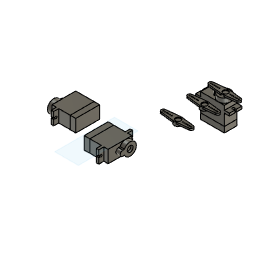
Chassis v8 (Autodesk Fusion 360 archive; units mm, degrees)
design "servo"
Autodesk Fusion 360 part; units mm, degrees
sketch "Sketch1" plane through (0, 0, 0) normal (0, 0, 1) x (1, 0, 0)
  line L0 (16, -5.9) -> (-16, -5.9)
  line L1 (-16, -5.9) -> (-16, 5.9)
  line L2 (-16, 5.9) -> (16, 5.9)
  line L3 (16, 5.9) -> (16, -5.9)
  line L4 (16, -5.9) -> (-16, 5.9) construction
  line L5 (-16, -5.9) -> (16, 5.9) construction
  line L6 (0, 0) -> (0, -5.9)
  circle A0 centre (-13.9, 0) radius 1.05
  line L7 (0, 0) -> (-16, 0)
  line L8 (-16, -0.575) -> (-14.7786, -0.575)
  line L9 (-16, 0.575) -> (-14.7786, 0.575)
  line L10 (16, -0.575) -> (14.7786, -0.575)
  circle A1 centre (13.9, 0) radius 1.05
  line L11 (16, 0.575) -> (14.7786, 0.575)
  dimension "d1" = 32
  dimension "d2" = 11.8
  dimension "d3" = 2.1
  dimension "d4" = 2.1
  dimension "d5" = 0.575
  constraint horizontal L0
  constraint perpendicular L0 L1
  constraint parallel L0 L2
  constraint parallel L1 L3
  constraint coincident L4 L6.start
  constraint coincident L5 L6.start
  constraint coincident L6.start L7.start
  constraint midpoint L0 L6.end
  constraint midpoint L1 L7.end
  constraint coincident L1 L8.start
  constraint coincident A0 L8.end
  constraint perpendicular L1 L8
  constraint coincident A0.centre L7
  constraint symmetric L7 L8.start L9.start
  constraint symmetric L7 L8.end L9.end
  constraint symmetric L6 A0 A1
  constraint symmetric L6 L8.start L10.start
  constraint symmetric L6 L8.end L10.end
  constraint symmetric L6 L9.start L11.start
  constraint symmetric L6 L9.end L11.end
  measures "d1" distance of L1.end L2.end
  measures "d2" distance of L0.end L1.end
  measures "d3" diameter of A0
  measures "d4" distance of L1 A0.centre
  measures "d5" distance of L7 L8
extrude "Extrude1" add sketch "Sketch1" along normal blind 2.3 contours L0 L1 L2 L3 L6 A0 L7 L9 L10 A1 L11 | L0 L1 L6 A0 L7 L8 makes body 1
sketch "Sketch2" plane through (0, 0, 2.3) normal (0, 0, 1) x (-1, 0, 0)
  line L0 (16, -0.575) -> (14.7786, -0.575)
  arc A0 (14.7786, 0.575) -> (14.7786, -0.575) centre (13.9, 0) ccw
  line L1 (14.7786, 0.575) -> (16, 0.575)
  line L2 (16, 0.575) -> (16, 5.9)
  line L3 (16, 5.9) -> (-16, 5.9)
  line L4 (-16, 5.9) -> (-16, 0.575)
  line L5 (-16, 0.575) -> (-14.7786, 0.575)
  arc A1 (-14.7786, -0.575) -> (-14.7786, 0.575) centre (-13.9, 0) ccw
  line L6 (-14.7786, -0.575) -> (-16, -0.575)
  line L7 (-16, -0.575) -> (-16, -5.9)
  line L8 (-16, -5.9) -> (16, -5.9)
  line L9 (16, -5.9) -> (16, -0.575)
  line L10 (11.25, -5.9) -> (-11.25, -5.9)
  line L11 (-11.25, -5.9) -> (-11.25, 5.9)
  line L12 (-11.25, 5.9) -> (11.25, 5.9)
  line L13 (11.25, 5.9) -> (11.25, -5.9)
  line L14 (11.25, -5.9) -> (-11.25, 5.9) construction
  line L15 (-11.25, -5.9) -> (11.25, 5.9) construction
  dimension "d8" = 22.5
  constraint horizontal L10
  constraint perpendicular L10 L11
  constraint parallel L10 L12
  constraint parallel L11 L13
  constraint coincident L14 origin
  constraint coincident L15 origin
  constraint coincident L3 L12.end
  measures "d8" distance of L11.end L12.end
extrude "Extrude2" add sketch "Sketch2" along normal blind 4.1 contours L3 L8 L10 L11 L12 L13 bodies 1
sketch "Sketch3" plane through (0, 0, 6.4) normal (0, 0, 1) x (-1, 0, 0)
  line L0 (11.25, 5.9) -> (-11.25, 5.9)
  line L1 (-11.25, 5.9) -> (-11.25, -5.9)
  line L2 (-11.25, -5.9) -> (11.25, -5.9)
  line L3 (11.25, -5.9) -> (11.25, 5.9)
  line L4 (0, 0) -> (-25, 0)
  line L5 (1.5394, 2.5) -> (-0.0028, 2.4935)
  line L6 (1.5394, -2.5) -> (-0.0028, -2.4935)
  arc A0 (1.5394, -2.5) -> (1.5394, 2.5) centre (1.55, 0) ccw
  arc A1 (-0.0028, 2.4935) -> (-0.0028, -2.4935) centre (-5.35, 0) ccw
  dimension "d11" = 5
  dimension "d12" = 6.9
  constraint coincident L4.start origin
  constraint parallel L0 L4
  constraint tangent L0 A1
  constraint tangent L1 A1
  constraint tangent L2 A1
  constraint tangent L5 A0
  constraint symmetric L4 L5.start L6.start
  measures "d11" diameter of A0
  measures "d12" distance of A1.centre A0.centre
extrude "Extrude3" add sketch "Sketch3" along normal blind 4.2 contours L5 L6 A0 A1 bodies 1
sketch "Sketch4" plane through (0, 0, 0) normal (0, 0, -1) x (1, 0, 0)
  line L0 (-14.7786, -0.575) -> (-16, -0.575)
  line L1 (-16, -0.575) -> (-16, -5.9)
  line L2 (-16, -5.9) -> (16, -5.9)
  line L3 (16, -5.9) -> (16, -0.575)
  line L4 (16, -0.575) -> (14.7786, -0.575)
  arc A0 (14.7786, 0.575) -> (14.7786, -0.575) centre (13.9, 0) ccw
  line L5 (14.7786, 0.575) -> (16, 0.575)
  line L6 (16, 0.575) -> (16, 5.9)
  line L7 (16, 5.9) -> (-16, 5.9)
  line L8 (-16, 5.9) -> (-16, 0.575)
  line L9 (-16, 0.575) -> (-14.7786, 0.575)
  arc A1 (-14.7786, -0.575) -> (-14.7786, 0.575) centre (-13.9, 0) ccw
  line L10 (11.25, -5.9) -> (11.25, 5.9)
  line L11 (11.25, 5.9) -> (-11.25, 5.9)
  line L12 (-11.25, 5.9) -> (-11.25, -5.9)
  line L13 (-11.25, -5.9) -> (11.25, -5.9)
extrude "Extrude4" add sketch "Sketch4" along normal blind 10.9 contours L2 L7 L10 L11 L12 L13 bodies 1
sketch "Sketch5" plane through (0, 0, -10.9) normal (0, 0, -1) x (1, 0, 0)
  line L0 (-11.25, -5.9) -> (11.25, -5.9)
  line L1 (11.25, -5.9) -> (11.25, 5.9)
  line L2 (11.25, 5.9) -> (-11.25, 5.9)
  line L3 (-11.25, 5.9) -> (-11.25, -5.9)
extrude "Extrude5" add sketch "Sketch5" along normal blind 5.3 draft 0.75 bodies 1
sketch "Sketch6" plane through (0, 0, 10.6) normal (0, 0, 1) x (-1, 0, 0)
  arc A0 (1.5394, -2.5) -> (1.5394, 2.5) centre (1.55, 0) ccw
  line L0 (1.5394, 2.5) -> (-0.0028, 2.4935)
  arc A1 (-0.0028, 2.4935) -> (-0.0028, -2.4935) centre (-5.35, 0) ccw
  line L1 (-0.0028, -2.4935) -> (1.5394, -2.5)
  circle A2 centre (-6.5803, -0.002) radius 3.58
  line L2 (-5.7591, -7.882) -> (-5.7591, 11) construction
  line L3 (-15, -0.002) -> (12, -0.002) construction
  line L4 (7.6454, 1.9853) -> (-6.1763, 3.5552)
  line L5 (7.6454, -1.9892) -> (-6.1763, -3.5591)
  circle A3 centre (7.4197, -0.002) radius 0.5
  circle A4 centre (5.8197, -0.002) radius 0.5
  circle A5 centre (4.2197, -0.002) radius 0.5
  circle A6 centre (2.6197, -0.002) radius 0.5
  circle A7 centre (1.0197, -0.002) radius 0.5
  circle A8 centre (-0.5803, -0.002) radius 0.5
  circle A9 centre (-10.9379, -0.002) radius 0.5
  circle A10 centre (-12.5379, -0.002) radius 0.5
  circle A11 centre (-14.1379, -0.002) radius 0.5
  circle A12 centre (-15.7379, -0.002) radius 0.5
  circle A13 centre (-17.3379, -0.002) radius 0.5
  circle A14 centre (-18.9379, -0.002) radius 0.5
  line L6 (-19.1636, -1.9892) -> (-5.3419, -3.5591)
  line L7 (-19.1636, 1.9853) -> (-5.3419, 3.5552)
  arc A15 (7.6454, -1.9892) -> (7.6454, 1.9853) centre (7.4197, -0.002) ccw
  arc A16 (-19.1636, 1.9853) -> (-19.1636, -1.9892) centre (-18.9379, -0.002) ccw
  dimension "d19" = 7.16
  dimension "d21" = 14
  dimension "d22" = 1
  dimension "d25" = -8
  dimension "d26" = 0
  constraint vertical L2
  constraint horizontal L3
  constraint coincident A2.centre L3
  constraint coincident A2 L4.end
  constraint tangent A2 L4
  constraint symmetric L3 L4.start L5.start
  constraint symmetric L3 L4.end L5.end
  constraint symmetric L2 L4.start L7.start
  constraint symmetric L2 L4.end L7.end
  constraint symmetric L2 L5.start L6.start
  constraint symmetric L2 L5.end L6.end
  constraint symmetric L2 A3 A14
  constraint symmetric L2 A4 A13
  constraint symmetric L2 A5 A12
  constraint symmetric L2 A6 A11
  constraint symmetric L2 A7 A10
  constraint symmetric L2 A8 A9
  measures "d19" diameter of A2
  measures "d21" distance of A2.centre A3.centre
  measures "d22" diameter of A3
extrude "Extrude6" add sketch "Sketch6" along normal blind 1.6 separate body contours A0 L0 A1 L1 A2 L4 L5 A5 L6 L7 | A0 L0 A1 L1 L4 L5 A5 A15 | A1 A9 L6 L7 A16 | A1 A2 A9 L6 L7 | A2 L6 | A2 L6 L7 | A2 L7 makes body 2
sketch "Sketch7" plane through (0, 0, 10.6) normal (0, 0, -1) x (1, 0, 0)
  circle A0 centre (18.9379, -0.002) radius 0.5
  circle A1 centre (17.3379, -0.002) radius 0.5
  circle A2 centre (-7.4197, -0.002) radius 0.5
  circle A3 centre (-5.8197, -0.002) radius 0.5
  circle A4 centre (10.9379, -0.002) radius 0.5
  circle A5 centre (15.7379, -0.002) radius 0.5
  circle A6 centre (14.1379, -0.002) radius 0.5
  circle A7 centre (-4.2197, -0.002) radius 0.5
  circle A8 centre (0.5803, -0.002) radius 0.5
  circle A9 centre (-1.0197, -0.002) radius 0.5
  circle A10 centre (-2.6197, -0.002) radius 0.5
  circle A11 centre (12.5379, -0.002) radius 0.5
  arc A12 (8.0932, 3.2427) -> (5.8336, 3.4993) centre (6.5803, -0.002) ccw
  line L0 (5.8336, 3.4993) -> (5.7591, 3.5078)
  line L1 (5.7591, 3.5078) -> (-7.6454, 1.9853)
  arc A13 (-7.6454, 1.9853) -> (-7.6454, -1.9892) centre (-7.4197, -0.002) ccw
  line L2 (-7.6454, -1.9892) -> (5.7591, -3.5117)
  line L3 (5.7591, -3.5117) -> (5.8336, -3.5032)
  arc A14 (5.8336, -3.5032) -> (8.0932, -3.2466) centre (6.5803, -0.002) ccw
  line L4 (8.0932, -3.2466) -> (19.1636, -1.9892)
  arc A15 (19.1636, -1.9892) -> (19.1636, 1.9853) centre (18.9379, -0.002) ccw
  line L5 (19.1636, 1.9853) -> (8.0932, 3.2427)
  circle A16 centre (6.5803, -0.002) radius 3.58
  constraint concentric A12 A16
  constraint tangent A12 A16
extrude "Extrude7" add sketch "Sketch7" along normal blind 1.83 contours A12 A14 A16 bodies 2
sketch "Sketch8" plane through (0, 0, 12.2) normal (0, 0, 1) x (-1, 0, 0)
  circle A0 centre (-18.9379, -0.002) radius 0.5
  circle A1 centre (-17.3379, -0.002) radius 0.5
  circle A2 centre (7.4197, -0.002) radius 0.5
  circle A3 centre (5.8197, -0.002) radius 0.5
  circle A4 centre (-10.9379, -0.002) radius 0.5
  circle A5 centre (-15.7379, -0.002) radius 0.5
  circle A6 centre (-14.1379, -0.002) radius 0.5
  circle A7 centre (4.2197, -0.002) radius 0.5
  circle A8 centre (-0.5803, -0.002) radius 0.5
  circle A9 centre (1.0197, -0.002) radius 0.5
  circle A10 centre (2.6197, -0.002) radius 0.5
  circle A11 centre (-12.5379, -0.002) radius 0.5
  arc A12 (-5.8336, 3.4993) -> (-8.0932, 3.2427) centre (-6.5803, -0.002) ccw
  line L0 (-8.0932, 3.2427) -> (-19.1636, 1.9853)
  arc A13 (-19.1636, 1.9853) -> (-19.1636, -1.9892) centre (-18.9379, -0.002) ccw
  line L1 (-19.1636, -1.9892) -> (-8.0932, -3.2466)
  arc A14 (-8.0932, -3.2466) -> (-5.8336, -3.5032) centre (-6.5803, -0.002) ccw
  line L2 (-5.8336, -3.5032) -> (-5.7591, -3.5117)
  line L3 (-5.7591, -3.5117) -> (7.6454, -1.9892)
  arc A15 (7.6454, -1.9892) -> (7.6454, 1.9853) centre (7.4197, -0.002) ccw
  line L4 (7.6454, 1.9853) -> (-5.7591, 3.5078)
  line L5 (-5.7591, 3.5078) -> (-5.8336, 3.4993)
  circle A16 centre (-6.5803, -0.002) radius 2.5
  dimension "d31" = 5
  constraint concentric A12 A16
  measures "d31" diameter of A16
extrude "Extrude8" cut sketch "Sketch8" against normal blind 0.8 contours A16 bodies 2
sketch "Sketch9" plane through (0, 0, 15) normal (0, 0, 1) x (-1, 0, 0)
  line L0 (0, 31.2947) -> (22.4, 31.2947)
  line L1 (22.4, 31.2947) -> (22.4, 87.7947)
  line L2 (22.4, 87.7947) -> (0, 87.7947)
  line L3 (0, 87.7947) -> (0, 31.2947)
copy_body "CopyPasteBodies1" bodies 1 2 makes body 3 makes body 4
move_body "Move1" bodies 3 4 to x (1, 0, 0) y (0, 1, 0) z (0, 0, 1) at (0, 25, 0)
copy_body "CopyPasteBodies2" bodies 3 4 makes body 5 makes body 6
move_body "Move2" bodies 5 6 to x (1, 0, 0) y (0, 1, 0) z (0, 0, 1) at (0, 20, 0)
move_body "Move3" bodies 1 to x (0, 1, 0) y (0, 0, 1) z (1, 0, 0) at (0.2, -14.9694, 29.7694)
sketch "Sketch10" plane through (10.8, 0, 0) normal (1, 0, 0) x (0, 1, 0)
  arc A0 (-16.5088, 32.2694) -> (-16.5088, 27.2694) centre (-16.5194, 29.7694) ccw
  line L0 (-16.5088, 27.2694) -> (-14.9666, 27.2759)
  arc A1 (-14.9666, 27.2759) -> (-14.9666, 32.2628) centre (-9.6194, 29.7694) ccw
  line L1 (-14.9666, 32.2628) -> (-16.5088, 32.2694)
  circle A2 centre (-9.6194, 29.7694) radius 2.75
  dimension "d34" = 5.5
  constraint concentric A1 A2
  measures "d34" diameter of A2
extrude "Extrude9" cut sketch "Sketch10" against normal blind 2 contours A2 bodies 1
move_body "Move4" bodies 1 to x (1, 0, 0) y (0, 1, 0) z (0, 0, 1) at (-5, -35, -20)
move_body "Move5" bodies 3 to x (0, -1, 0) y (0, 0, 1) z (-1, 0, 0) at (-47.2, -6.9694, -5.2306)
sketch "Sketch11" plane through (-57.8, 0, 0) normal (-1, 0, 0) x (0, -1, 0)
  arc A0 (5.4299, 22.2694) -> (5.4299, 17.2694) centre (5.4194, 19.7694) ccw
  line L0 (5.4299, 17.2694) -> (6.9722, 17.2759)
  arc A1 (6.9722, 17.2759) -> (6.9722, 22.2628) centre (12.3194, 19.7694) ccw
  line L1 (6.9722, 22.2628) -> (5.4299, 22.2694)
  circle A2 centre (12.3194, 19.7694) radius 2.75
  dimension "d37" = 5.5
  constraint concentric A1 A2
  measures "d37" diameter of A2
extrude "Extrude10" cut sketch "Sketch11" against normal blind 2 contours A2 bodies 3
move_body "Move6" bodies 3 to x (1, 0, 0) y (0, 1, 0) z (0, 0, 1) at (-8, -33, -10)
sketch "Sketch12" plane through (-57.5, 0, 0) normal (-1, 0, 0) x (0, -1, 0)
  line L0 (28.7194, 3.8694) -> (28.7194, 15.6694)
  line L1 (28.7194, 15.6694) -> (23.9694, 15.6694)
  line L2 (23.9694, 15.6694) -> (23.9694, 10.3444)
  line L3 (23.9694, 10.3444) -> (25.1908, 10.3444)
  arc A0 (25.1908, 9.1944) -> (25.1908, 10.3444) centre (26.0694, 9.7694) ccw
  line L4 (25.1908, 9.1944) -> (23.9694, 9.1944)
  line L5 (23.9694, 9.1944) -> (23.9694, 3.8694)
  line L6 (23.9694, 3.8694) -> (28.7194, 3.8694)
  line L7 (23.9694, 15.6694) -> (28.7194, 15.6694)
  line L8 (28.7194, 15.6694) -> (28.7194, 3.8694)
  line L9 (28.7194, 3.8694) -> (23.9694, 3.8694)
  line L10 (23.9694, 3.8694) -> (23.9694, 15.6694)
  constraint horizontal L7
  constraint vertical L8
  constraint horizontal L9
  constraint vertical L10
  constraint coincident L0.start L6.end
  constraint coincident L1.end L2.start
extrude "Extrude11" cut sketch "Sketch12" against normal through all contours L0 L1 L2 L3 A0 L4 L5 L6 L7 L8 L9 L10 bodies 3
